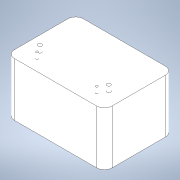
# Autodesk Inventor part: Battery
Saved by Autodesk Inventor 2022 (Build 260153000, 153)
## iProperties
Created: 2022-08-12
Part Number: Battery
Material: Generic
Document SubType Name: Modeling
Designer: Alok
Density: 1 g/cm^3
Appearance: Default
Author: Alok
Autodesk Inventor part; units mm, degrees
ref_plane "YZ Plane" through (0, 0, 0) normal (1, 0, 0) x (0, 1, 0)
ref_plane "XZ Plane" through (0, 0, 0) normal (0, 1, 0) x (-1, 0, 0)
ref_plane "XY Plane" through (0, 0, 0) normal (0, 0, 1) x (1, 0, 0)
sketch "Sketch1" plane through (0, 0, 0) normal (0, 1, 0) x (-1, 0, 0)
  line L0 (127.5, 90) -> (-127.5, 90)
  line L1 (-127.5, 90) -> (-127.5, -90)
  line L2 (-127.5, -90) -> (127.5, -90)
  line L3 (127.5, -90) -> (127.5, 90)
  line L4 (127.5, 90) -> (-127.5, -90) construction
  line L5 (-127.5, 90) -> (127.5, -90) construction
  point P0 (0, 0)
  dimension "d0" = 255
  dimension "d1" = 180
  constraints: 12 end point, 2 midpoint, 2 parallel, 1 horizontal, 1 perpendicular
  measures "d0" distance of L2.end L1.end
  measures "d1" distance of L1.end L0.end
extrude "Extrusion1" add sketch "Sketch1" along normal blind 140
fillet "Face Fillet1" radius 20 1 edges at (127.5, 70, 90)
fillet "Face Fillet2" radius 20 1 edges at (127.5, 70, -90)
fillet "Face Fillet3" radius 20 1 edges at (-127.5, 70, -90)
fillet "Face Fillet4" radius 20 1 edges at (-127.5, 70, 90)
sketch "Sketch2" plane through (0, 140, 0) normal (0, 1, 0) x (1, 0, 0)
  line L0 (0, 0) -> (0, -90)
  line L1 (-107.5, -90) -> (107.5, -90) projected
  line L2 (-127.5, 70) -> (-127.5, -70) projected
  circle A0 centre (-90, -40.8457) radius 5
  circle A1 centre (-77.8212, -60.1893) radius 3
  dimension "d9" = 10
  dimension "d10" = 6
  constraints: 2 centre point, 2 end point, 1 midpoint
  measures "d9" diameter of A0
  measures "d10" diameter of A1
extrude "Extrusion2" add sketch "Sketch2" along normal blind 15
mirror "Mirror1" about plane through (0, 0, 0) normal (1, 0, 0) of "Extrusion2"
body "Solid1"
